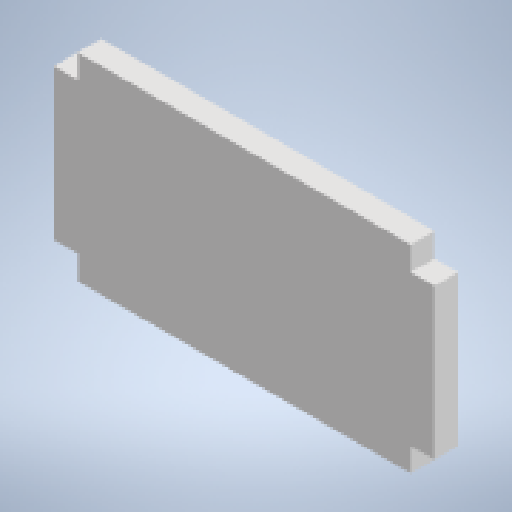
# Autodesk Inventor part: front support
Saved by Autodesk Inventor 2023 (Build 270158000, 158)
## iProperties
Created: 2023-11-14
Part Number: front support
Material: Generic
Document SubType Name: Modeling
Designer: Nate
Density: 1 g/cm^3
Appearance: Default
Author: Nate
Autodesk Inventor part; units mm, degrees
ref_plane "YZ Plane" through (0, 0, 0) normal (1, 0, 0) x (0, 1, 0)
ref_plane "XZ Plane" through (0, 0, 0) normal (0, 1, 0) x (-1, 0, 0)
ref_plane "XY Plane" through (0, 0, 0) normal (0, 0, 1) x (1, 0, 0)
sketch "Sketch1" plane through (0, 0, 0) normal (0, 0, 1) x (1, 0, 0)
  line L0 (0, 0) -> (50.8, 0)
  line L1 (50.8, 0) -> (50.8, 20.066)
  line L2 (50.8, 20.066) -> (0, 20.066)
  line L3 (0, 20.066) -> (0, 0)
  line L4 (3.175, 20.066) -> (47.625, 20.066)
  line L5 (47.625, 20.066) -> (47.625, 23.241)
  line L6 (47.625, 23.241) -> (3.175, 23.241)
  line L7 (3.175, 23.241) -> (3.175, 20.066)
  line L8 (3.175, 0) -> (47.625, 0)
  line L9 (47.625, 0) -> (47.625, -3.175)
  line L10 (47.625, -3.175) -> (3.175, -3.175)
  line L11 (3.175, -3.175) -> (3.175, 0)
  point P0 (47.625, -1.5875)
  dimension "d0" = 3.175
  dimension "d1" = 3.175
  dimension "d2" = 3.175
  dimension "d3" = 3.175
  dimension "d4" = 3.175
  dimension "d5" = 3.175
  dimension "d6" = 44.45
  dimension "d7" = 20.066
  constraints: 24 end point, 6 parallel, 3 horizontal, 3 perpendicular, 3 point on line, 1 midpoint
  measures "d0" distance between parallel lines of L0 L10
  measures "d1" distance between parallel lines of L3 L11
  measures "d2" distance from line of L1 point (47.625, -1.587)
  measures "d3" distance between parallel lines of L3 L7
  measures "d4" distance between parallel lines of L1 L5
  measures "d5" distance between parallel lines of L2 L6
  measures "d6" distance between parallel lines of L9 L11
  measures "d7" distance between parallel lines of L2 L0
extrude "Extrusion1" add sketch "Sketch1" along normal blind 3.175
body "Solid1"
